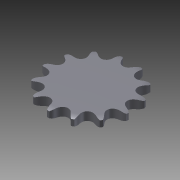
# Autodesk Inventor part: Roller Chain Sprocket1
Saved by Autodesk Inventor 2014 (Build 180170000, 170)
## iProperties
Created: 2013-07-16
Part Number: Roller Chain Sprocket1
Material: Steel
Document SubType Name: Modeling
Designer: Mill
Density: 1 g/cm^3
Appearance: Steel
CustomPartVersion: 1
Author: Mill
Autodesk Inventor part; units mm, degrees
ref_plane "YZ Plane" through (0, 0, 0) normal (1, 0, 0) x (0, 1, 0)
ref_plane "XZ Plane" through (0, 0, 0) normal (0, 1, 0) x (-1, 0, 0)
sketch "Theoretical Tooth Profile" plane through (0, 0, 0) normal (0, 0, 1) x (1, 0, 0)
  circle A0 centre (0, 0) radius 26.534 construction
  line L0 (0, 0) -> (0, 26.534) construction
  line L1 (0, 0) -> (12.331, 23.4947) construction
  circle A1 centre (0, 0) radius 29.573
  arc A2 (-3.0227, 24.032) -> (3.0227, 24.032) centre (0, 26.534) ccw
  line L2 (0, 26.534) -> (12.331, 23.4947) construction
  line L3 (0, 26.534) -> (4.7884, 30.4975) construction
  line L4 (4.7884, 30.4975) -> (-4.3312, 26.0647) construction
  arc A3 (6.3066, 28.8927) -> (4.6829, 26.7883) centre (10.5619, 23.9307) ccw
  arc A4 (-4.6829, 26.7883) -> (-6.3066, 28.8927) centre (-10.5619, 23.9307) ccw
  line L5 (-10.5619, 23.9307) -> (-4.6829, 26.7883) construction
  arc A5 (-4.3312, 26.0647) -> (-3.0227, 24.032) centre (4.7884, 30.4975) ccw
  line L6 (-4.3312, 26.0647) -> (-4.6829, 26.7883)
  arc A6 (3.0227, 24.032) -> (4.3312, 26.0647) centre (-4.7884, 30.4975) ccw
  line L7 (4.6829, 26.7883) -> (4.3312, 26.0647)
  line L8 (0, 0) -> (7.0773, 28.7136) construction
  point P0 (6.1655, 25.0143)
  dimension "d0" = 53.068
  dimension "d2" = 27.692
  dimension "d3" = 3.9238
  dimension "d10" = 129.615
  dimension "d11" = 13.692
  dimension "d12" = 6.216
  dimension "d13" = 10.1398
  dimension "d14" = 10.878
  dimension "d23" = 3.81
  constraints: 18 end point, 15 point on circle, 7 centre point, 3 coincident, 3 point on line, 3 symmetric about line, 3 tangent, 1 equal radius, 1 midpoint, 1 parallel, 1 vertical, 1 other
  measures "d0" diameter of A0
  measures "d2" angle of L1 L0
  measures "d3" radius of A2
  measures "d10" angle of L3 L0
  measures "d11" angle of L4 L3
  measures "d12" distance of L2.start L3.end
  measures "d13" distance of L3.end L4.end
  measures "d14" distance of A3.centre L0.end
  measures "d23" distance from line of L8.end L2
sketch "Tooth Profile" plane through (0, 0, 0) normal (0, 0, 1) x (1, 0, 0)
  arc A0 (-3.5995, 24.9718) -> (3.5995, 24.9718) centre (0, 26.534) ccw
  arc A1 (6.1801, 28.92) -> (3.5995, 24.9718) centre (16.4292, 19.4035) ccw
  arc A2 (-3.5995, 24.9718) -> (-6.1801, 28.92) centre (-16.4292, 19.4035) ccw
  line L0 (0, 0) -> (0, 26.534) construction
  line L1 (0, 26.534) -> (3.5995, 24.9718) construction
  line L2 (0, 26.534) -> (-3.5995, 24.9718) construction
  circle A3 centre (0, 0) radius 29.573 projected
  dimension "d44" = 133.077
  dimension "d45" = 13.986
  dimension "d46" = 3.9238
  constraints: 9 point on circle, 6 end point, 3 centre point, 2 tangent, 1 coincident, 1 equal radius, 1 vertical, 1 other
  measures "d44" angle of L2 L1
  measures "d45" radius of A1
  measures "d46" radius of A0
sketch "Section Profile" plane through (0, 0, 0) normal (1, 0, 0) x (0, 1, 0)
  line L0 (29.573, 0) -> (-29.573, 0) projected
  line L1 (16.3018, 2.9063) -> (-16.3018, 2.9063)
  line L2 (-16.3018, 2.9063) -> (-16.3018, -2.9062)
  line L3 (-16.3018, -2.9062) -> (16.3018, -2.9062)
  line L4 (16.3018, -2.9062) -> (16.3018, 2.9063)
  line L5 (16.3018, 2.9062) -> (29.573, 2.9062) construction
  line L6 (29.573, 2.9062) -> (29.573, -2.9062) construction
  line L7 (29.573, -2.9062) -> (16.3018, -2.9062) construction
  line L8 (16.3018, -2.9062) -> (16.3018, 2.9062)
  arc A0 (29.573, 2.1443) -> (25.24, 2.9063) centre (25.24, -9.7937) ccw
  arc A1 (25.24, -2.9063) -> (29.573, -2.1443) centre (25.24, 9.7937) ccw
  line L9 (25.24, 2.9063) -> (0, 2.9062)
  line L10 (0, 2.9062) -> (0, -2.9062)
  line L11 (0, -2.9062) -> (25.24, -2.9063)
  line L12 (0, 2.9062) -> (0, -2.9062)
  line L13 (29.573, 2.1443) -> (29.573, -2.1443)
  point P0 (0, 0)
  point P1 (0, 0)
  dimension "d30" = 5.8125
  dimension "d31" = 32.6035
  dimension "d32" = 5.8125
  dimension "d33" = 0.762
  dimension "d34" = 12.7
  dimension "d43" = 2.9062
  constraints: 26 end point, 7 midpoint, 5 perpendicular, 4 parallel, 4 point on circle, 3 point on line, 3 symmetric about line, 2 centre point, 2 horizontal, 2 tangent, 1 collinear, 1 other
  measures "d30" distance between parallel lines of L7 L5
  measures "d31" distance between parallel lines of L2 L4
  measures "d32" distance between parallel lines of L3 L1
  measures "d33" distance from line of L13.start L5
  measures "d34" radius of A0
  measures "d43" distance between parallel lines of L3 L0
revolve "Shroud" add sketch "Section Profile" angle 360 about axis through (0, 0, 2.9062) along (0, 0, -1) contours L10 L3 L2 L0 | L0 L2 L1 L10
revolve "Strand" add sketch "Section Profile" angle 360 about axis through (0, 0, 2.9062) along (0, 0, -1) contours L13 A1 L11 L4 L0 | L0 L4 L9 A0 L13 | L4 L3 L10 L0 | L0 L10 L1 L4
pattern_of_one "Strand Pattern"
extrude "Theoretical Tooth" cut sketch "Theoretical Tooth Profile" along normal through all both and the other way through all contours A3 L7 A6 A2 A5 L6 A4 A1 picked at (0, 27.2015)
extrude "Tooth" [suppressed]
pattern_circular "Tooth Pattern" count 13 over 360 about axis through (0, 0, -10) along (0, 0, 1) of "Theoretical Tooth"
ref_plane "Timing Plane" through (0, 26.534, 0) normal (1, 0, 0) x (0, 1, 0)
equation "\"d3\" = 0.5 * da_Dr + da_SC"
equation "\"d12\" = 0.8 * da_Dr"
equation "\"d13\" = 1.3 * da_Dr + da_SC"
equation "\"d14\" = 1.4 * da_Dr"
equation "\"d23\" = da_Ha"
equation "\"d44\" = da_Alfa"
equation "\"d45\" = da_Re"
equation "\"d46\" = da_Ri"
equation "\"d30\" = da_Bf"
equation "\"d31\" = da_Ds"
equation "\"d32\" = da_Bs"
equation "\"d33\" = da_Ba"
equation "\"d34\" = da_Rx"
equation "\"d40\" = da_pt"
equation "\"form_type\" = 0"
equation "\"da_p\" = 12.7"
equation "\"da_Dr\" = 7.77"
equation "\"da_SC\" = 0.03885"
equation "\"da_Ha\" = 3.81"
equation "\"da_pt\" = 13.92"
equation "\"da_Bf\" = 5.8125"
equation "\"da_Ba\" = 0.762"
equation "\"da_Rx\" = 12.7"
equation "\"da_Ra\" = 0.508"
equation "\"da_Bs\" = 5.8125"
equation "\"da_Ds\" = 32.60353"
equation "\"da_Re\" = 13.986"
equation "\"da_Ri\" = 3.92385"
equation "\"da_Alfa\" = 133.077deg"
body "Solid1"
